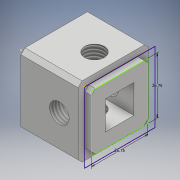
# Autodesk Inventor part: cuvette holder blockBASE_with_bottom_drain
Saved by Autodesk Inventor 2017 (Build 210142000, 142)
## iProperties
Created: 2018-08-10
Part Number: cuvette holder blockBASE_with_bottom_drain
Material: Generic
Document SubType Name: Modeling
Designer: qwertyuiop1
Density: 1 g/cm^3
Appearance: Default
Author: qwertyuiop1
Autodesk Inventor part; units mm, degrees
ref_plane "YZ Plane" through (0, 0, 0) normal (1, 0, 0) x (0, 1, 0)
ref_plane "XZ Plane" through (0, 0, 0) normal (0, 1, 0) x (-1, 0, 0)
ref_plane "XY Plane" through (0, 0, 0) normal (0, 0, 1) x (1, 0, 0)
sketch "Sketch1" plane through (0, 0, 0) normal (1, 0, 0) x (0, 1, 0)
  line L0 (0, 0) -> (33.25, 0)
  line L1 (33.25, 0) -> (33.25, -33.25)
  line L2 (33.25, -33.25) -> (0, -33.25)
  line L3 (0, -33.25) -> (0, 0)
  dimension "d0" = 33.25
  dimension "d1" = 33.25
  constraints: 8 end point, 2 parallel, 1 horizontal, 1 perpendicular
  measures "d0" distance of L1.end L2.end
  measures "d1" distance of L0.end L1.end
extrude "Extrusion1" add sketch "Sketch1" along normal blind 30
sketch "Sketch2" plane through (30, 0, 0) normal (1, 0, 0) x (0, 0, -1)
  line L0 (3.25, 3.25) -> (30, 3.25)
  line L1 (30, 3.25) -> (30, 30)
  line L2 (30, 30) -> (3.25, 30)
  line L3 (3.25, 30) -> (3.25, 3.25)
  point P0 (0, 0)
  dimension "d4" = 26.75
  dimension "d5" = 26.75
  constraints: 8 end point, 2 parallel, 1 horizontal, 1 perpendicular
  measures "d4" distance of L2.end L1.end
  measures "d5" distance of L1.end L0.end
sketch "Sketch3" plane through (30, 0, 0) normal (1, 0, 0) x (0, 0, -1)
  line L0 (33.25, 0) -> (33.25, 33.25) projected
  line L1 (0, 0) -> (33.25, 0)
  line L2 (33.25, 0) -> (33.25, 33.25)
  line L3 (33.25, 33.25) -> (0, 33.25)
  line L4 (0, 33.25) -> (0, 0)
  constraints: 8 end point, 2 parallel, 1 horizontal, 1 perpendicular
sketch "Sketch4" plane through (30, 0, 0) normal (1, 0, 0) x (0, 0, -1)
  line L0 (3.25, 3.25) -> (30, 3.25)
  line L1 (30, 3.25) -> (30, 30)
  line L2 (30, 30) -> (3.25, 30)
  line L3 (3.25, 30) -> (3.25, 3.25)
  line L4 (0, 33.25) -> (0, 0) projected
  line L5 (33.25, 0) -> (33.25, 33.25) projected
  line L6 (0, 0) -> (33.25, 0)
  line L7 (33.25, 0) -> (33.25, 33.25)
  line L8 (33.25, 33.25) -> (0, 33.25)
  line L9 (0, 33.25) -> (0, 0)
  dimension "d6" = 26.75
  dimension "d7" = 26.75
  constraints: 16 end point, 4 parallel, 2 horizontal, 2 perpendicular
  measures "d6" distance of L2.end L1.end
  measures "d7" distance of L1.end L0.end
extrude "Extrusion2" cut sketch "Sketch4" against normal blind 3
chamfer "Chamfer1" distance 1.875 angle 45 8 edges at (13.5, 33.25, 0) (13.5, 33.25, -33.25) (28.5, 30, -3.25) (28.5, 30, -30) (28.5, 3.25, -3.25) (13.5, 0, 0) (28.5, 3.25, -30) (13.5, 0, -33.25)
sketch "Sketch5" plane through (30, 0, 0) normal (1, 0, 0) x (0, 0, -1)
  line L0 (9.875, 9.875) -> (23.375, 9.875)
  line L1 (23.375, 9.875) -> (23.375, 23.375)
  line L2 (23.375, 23.375) -> (9.875, 23.375)
  line L3 (9.875, 23.375) -> (9.875, 9.875)
  line L4 (28.125, 30) -> (5.125, 30) projected
  line L5 (30, 5.125) -> (30, 28.125) projected
  line L6 (3.25, 3.25) -> (30, 3.25)
  line L7 (30, 3.25) -> (30, 30)
  line L8 (30, 30) -> (3.25, 30)
  line L9 (3.25, 30) -> (3.25, 3.25)
  point P0 (0, 0)
  dimension "d13" = 13.5
  dimension "d14" = 13.5
  dimension "d15" = 6.625
  dimension "d16" = 6.625
  constraints: 16 end point, 4 parallel, 2 horizontal, 2 perpendicular
  measures "d13" distance of L2.end L1.end
  measures "d14" distance of L1.end L0.end
  measures "d15" distance between parallel lines of L4 L2
  measures "d16" distance between parallel lines of L5 L1
extrude "Extrusion3" cut sketch "Sketch5" against normal blind 26.75 contours L3 L2 L1 L0
sketch "Sketch6" plane through (0, 1.875, 0) normal (0, 0, 1) x (1, 0, 0)
  point P0 (0, -1.875)
sketch "Sketch7" plane through (0, 1.875, 0) normal (0, 0, 1) x (1, 0, 0)
  circle A0 centre (18.125, 14.75) radius 4.625
  point P0 (0, -1.875)
  dimension "d19" = 9.25
  constraints: 1 centre point
  measures "d19" diameter of A0
extrude "Extrusion4" cut sketch "Sketch7" against normal blind 33.25
sketch "Sketch8" plane through (0, 0, -31.375) normal (0, -1, 0) x (1, 0, 0)
  circle A0 centre (18.125, 14.75) radius 4.625
  point P0 (0, 31.375)
  dimension "d22" = 9.25
  constraints: 1 centre point
  measures "d22" diameter of A0
extrude "Extrusion5" cut sketch "Sketch8" against normal blind 33.25
thread "Thread1" size "M10x1.5" class "6H" standard "ANSI Metric M Profile" full length
thread "Thread2" size "M10x1.5" class "6H" standard "ANSI Metric M Profile" full length
thread "Thread3" size "M10x1.5" class "6H" standard "ANSI Metric M Profile" full length
thread "Thread4" size "M10x1.5" class "6H" standard "ANSI Metric M Profile" full length
sketch "Sketch9" plane through (0, 0, 0) normal (-1, 0, 0) x (0, 0, 1)
  circle A0 centre (-16.625, 16.625) radius 4.625
  point P0 (0, 0)
  dimension "d33" = 9.25
  constraints: 1 centre point
  measures "d33" diameter of A0
extrude "Extrusion6" cut sketch "Sketch9" against normal blind 10
thread "Thread5" size "M10x1.5" class "6H" standard "ANSI Metric M Profile" full length
body "Solid1"
